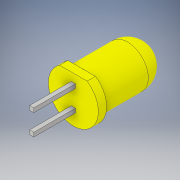
# Autodesk Inventor part: LED_5mm_Gelb
Saved by Autodesk Inventor 2018 (Build 220112000, 112)
## iProperties
Created: 2019-08-04
Part Number: LED_5mm_Gelb
Material: Generisch
Document SubType Name: Modeling
Designer: Admin
Density: 1 g/cm^3
Appearance: Vorgabe
Author: Admin
Autodesk Inventor part; units mm, degrees
ref_plane "YZ Plane" through (0, 0, 0) normal (1, 0, 0) x (0, 1, 0)
ref_plane "XZ Plane" through (0, 0, 0) normal (0, 1, 0) x (-1, 0, 0)
ref_plane "XY Plane" through (0, 0, 0) normal (0, 0, 1) x (1, 0, 0)
sketch "Skizze1" plane through (0, 0, 0) normal (0, 1, 0) x (-1, 0, 0)
  circle A0 centre (0, 0) radius 2.5
  dimension "d0" = 5
  constraints: 1 centre point, 1 coincident
  measures "d0" diameter of A0
extrude "Höhe" add sketch "Skizze1" along normal blind 8
fillet "Radius_Kopf" radius 2.5 1 edges at (2.5, 8, 0)
sketch "Skizze2" plane through (0, 0, 0) normal (0, -1, 0) x (1, 0, 0)
  arc A0 (-1.6583, 2.5) -> (1.6583, 2.5) centre (0, 0) ccw
  line L0 (-1.6583, 2.5) -> (1.6583, 2.5)
  circle A1 centre (0, 0) radius 2.5 projected
  dimension "d4" = 6
  constraints: 2 end point, 2 point on circle, 1 centre point, 1 coincident, 1 horizontal, 1 tangent
  measures "d4" diameter of A0
extrude "Kante" add sketch "Skizze2" along normal blind 1 contours A1 | L0 A0
sketch "Skizze3" plane through (0, -1, 0) normal (0, -1, 0) x (1, 0, 0)
  circle A0 centre (0, 0) radius 2.5 construction
  line L0 (0, 2.5) -> (0, -3) construction
  arc A1 (-1.6583, 2.5) -> (1.6583, 2.5) centre (0, 0) ccw construction
  line L1 (-2.5, 0) -> (2.5, 0) construction
  line L2 (-0.25, 1.52) -> (0.25, 1.52)
  line L3 (0.25, 1.52) -> (0.25, 1.02)
  line L4 (0.25, 1.02) -> (-0.25, 1.02)
  line L5 (-0.25, 1.02) -> (-0.25, 1.52)
  line L6 (-0.25, 1.27) -> (0.25, 1.27) construction
  line L7 (-0.25, -1.52) -> (0.25, -1.52)
  line L8 (0.25, -1.52) -> (0.25, -1.02)
  line L9 (0.25, -1.02) -> (-0.25, -1.02)
  line L10 (-0.25, -1.02) -> (-0.25, -1.52)
  point P0 (0, 1.27)
  point P1 (0, -1.27)
  dimension "d7" = 2.54
  dimension "d8" = 0.5
  dimension "d9" = 0.5
  constraints: 22 end point, 5 symmetric about line, 4 midpoint, 4 point on circle, 3 point on line, 2 horizontal, 2 parallel, 1 coincident, 1 perpendicular, 1 vertical, 1 other
  measures "d7" distance of point (0, -1.27) point (0, 1.27)
  measures "d8" distance between parallel lines of L4 L2
  measures "d9" distance between parallel lines of L3 L5
extrude "Pin" add sketch "Skizze3" along normal blind 5
